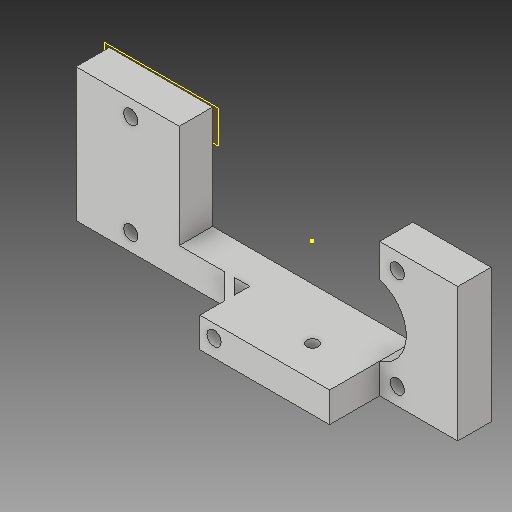
# Autodesk Inventor part: Aide_rotate
Saved by Autodesk Inventor 2017 (Build 210142000, 142)
## iProperties
Part Number: Aide_rotate
Material: Générique
Document SubType Name: Modeling
Designer: Thomas
Density: 1 g/cm^3
Appearance: Par défaut
Author: Thomas
Autodesk Inventor part; units mm, degrees
ref_plane "YZ Plane" through (0, 0, 0) normal (1, 0, 0) x (0, 1, 0)
ref_plane "XZ Plane" through (0, 0, 0) normal (0, 1, 0) x (-1, 0, 0)
ref_plane "XY Plane" through (0, 0, 0) normal (0, 0, 1) x (1, 0, 0)
sketch "Esquisse1" plane through (0, 0, 0) normal (0, 0, 1) x (1, 0, 0)
  line L0 (30.1547, 20.0742) -> (30.1547, 11.0742) projected
  line L1 (30.1547, 11.0742) -> (49.0652, 11.0742) projected
  line L2 (49.0652, 11.0742) -> (49.0652, -11.0742) projected
  line L3 (49.0652, -11.0742) -> (-60.9348, -11.0742) projected
  line L4 (-60.9348, -11.0742) -> (-60.9348, -20.0742) projected
  line L5 (-60.9348, -20.0742) -> (53.6264, -20.0742) projected
  line L6 (53.6264, -20.0742) -> (53.6264, 20.0742) projected
  line L7 (53.6264, 20.0742) -> (30.1547, 20.0742) projected
  circle A0 centre (35.4871, 15.0742) radius 2.15 projected
  circle A1 centre (-44.5129, -14.9258) radius 2.15 projected
  circle A2 centre (-4.5129, -14.9258) radius 2.15 projected
  circle A3 centre (35.4871, -14.9258) radius 2.15 projected
  line L8 (30.1547, 11.0742) -> (30.1547, -11.0742)
  point P0 (0, 0)
  constraints: 2 end point, 1 perpendicular, 1 point on line
extrude "Extrusion1" add sketch "Esquisse1" along normal blind 10
sketch "Esquisse2" plane through (0, 0, 10) normal (0, 0, 1) x (1, 0, 0)
  circle A0 centre (35.4871, -14.9258) radius 2.15 projected
  circle A1 centre (-4.5129, -14.9258) radius 2.15 projected
  circle A2 centre (-44.5129, -14.9258) radius 2.15 projected
  circle A3 centre (35.4871, 15.0742) radius 2.15 projected
  line L0 (30.1547, 20.0742) -> (30.1547, -11.0742) projected
  line L1 (30.1547, -11.0742) -> (-60.9348, -11.0742) projected
  line L2 (-60.9348, -11.0742) -> (-60.9348, -20.0742) projected
  line L3 (-60.9348, -20.0742) -> (53.6264, -20.0742) projected
  line L4 (53.6264, -20.0742) -> (53.6264, 20.0742) projected
  line L5 (53.6264, 20.0742) -> (30.1547, 20.0742) projected
  line L6 (-60.9348, -20.0742) -> (53.6264, -20.0742) projected
  line L7 (30.1547, -20.0742) -> (30.1547, -11.0742)
  line L8 (-60.9348, -20.0742) -> (53.6264, -20.0742) projected
  line L9 (-8.7922, -20.0742) -> (-8.7922, -11.0742)
  line L10 (30.1547, -11.0742) -> (-60.9348, -11.0742) projected
  point P0 (0, 0)
  constraints: 4 end point, 3 point on line, 2 perpendicular
extrude "Extrusion2" add sketch "Esquisse2" along normal blind 15 contours L7 L3 L9 L1
sketch "Esquisse3" plane through (-60.9348, -11.0742, 0) normal (0, 1, 0) x (1, 0, 0)
  line L0 (91.0895, 0) -> (91.0895, -10) projected
  line L1 (91.0895, 0) -> (0, 0) projected
  line L2 (0, 0) -> (0, -10) projected
  line L3 (52.1426, -10) -> (0, -10) projected
  line L4 (52.1426, -10) -> (52.1426, -25) projected
  line L5 (91.0895, -25) -> (52.1426, -25) projected
  line L6 (91.0895, -10) -> (91.0895, -25) projected
  line L7 (91.0895, 0) -> (0, 0) projected
  line L8 (30.9674, 0) -> (30.9674, -10)
  point P0 (60.9348, 0)
  constraints: 2 end point, 2 point on line, 1 perpendicular
extrude "Extrusion3" add sketch "Esquisse3" along normal blind 31 contours L8 L3 L2 L1
ref_plane "Plan de construction1" through (0, 0, 0) normal (0, 0, 1) x (1, 0, 0)
sketch "Esquisse4" plane through (0, 0, 0) normal (0, 0, 1) x (1, 0, 0)
  point P0 (0, 0)
sketch "Esquisse5" plane through (0, 0, 0) normal (0, 0, 1) x (1, 0, 0)
  circle A0 centre (-44.5129, 15.0742) radius 2.15 projected
  point P0 (0, 0)
extrude "Extrusion4" cut sketch "Esquisse5" along normal blind 31
sketch "Esquisse6" plane through (-8.7922, -11.0742, 25) normal (0, 1, 0) x (1, 0, 0)
  line L0 (6.4293, 0) -> (2.1293, 0) projected
  line L1 (4.2793, 0) -> (4.2793, 25) construction
  line L2 (2.1293, 25) -> (6.4293, 25) projected
  line L3 (4.2793, 25) -> (4.2793, 9.5)
  line L4 (4.2793, 9.5) -> (24.2793, 9.5) construction
  circle A0 centre (24.2793, 9.5) radius 1.75
  point P0 (8.7922, 25)
  dimension "d8" = 15.5
  dimension "d9" = 20
  dimension "d10" = 3.5
  constraints: 6 end point, 2 midpoint, 1 centre point, 1 coincident, 1 perpendicular, 1 point on line
  measures "d8" distance of L1.end L3.end
  measures "d9" distance of L3.end L4.end
  measures "d10" diameter of A0
extrude "Extrusion5" cut sketch "Esquisse6" against normal blind 10
sketch "Esquisse7" plane through (0, 0, 10) normal (0, 0, 1) x (1, 0, 0)
  line L0 (30.1547, -11.0742) -> (30.1547, -20.0742) projected
  line L1 (30.1547, 20.0742) -> (30.1547, -11.0742) projected
  arc A0 (30.1547, -11.0742) -> (30.1547, 10.0925) centre (27.156, -0.4909) ccw
  line L2 (30.1547, -11.0742) -> (-29.9674, -11.0742) projected
  line L3 (30.1547, -11.0742) -> (30.1547, 10.0925)
  point P0 (0, 0)
  dimension "d13" = 11
  constraints: 2 end point, 2 point on circle, 1 centre point, 1 collinear, 1 point on line
  measures "d13" radius of A0
extrude "Extrusion6" cut sketch "Esquisse7" against normal blind 10
sketch "Esquisse8" plane through (-8.7922, -11.0742, 25) normal (0, 1, 0) x (1, 0, 0)
  line L0 (0, 15) -> (0, 0) projected
  line L1 (0, 7.5) -> (-7.5714, 15)
  line L2 (0, 15) -> (-21.1752, 15) projected
  line L3 (0, 10.3151) -> (-4.7295, 15)
  point P0 (8.7922, 25)
  dimension "d16" = 2
  constraints: 4 end point, 3 point on line, 1 midpoint, 1 parallel
  measures "d16" distance between parallel lines of L1 L3
extrude "Extrusion7" add sketch "Esquisse8" against normal blind 9 contours L0 L1 L2 L3
